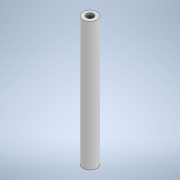
# Autodesk Inventor part: soprye para base bobinas
Saved by Autodesk Inventor 2020 (Build 240168000, 168)
## iProperties
Created: 2022-10-18
Part Number: soprye para base bobinas
Material: Genérico
Document SubType Name: Modeling
Designer: General
Density: 1 g/cm^3
Appearance: Valor por defecto
Author: General
Autodesk Inventor part; units mm, degrees
ref_plane "YZ Plane" through (0, 0, 0) normal (1, 0, 0) x (0, 1, 0)
ref_plane "XZ Plane" through (0, 0, 0) normal (0, 1, 0) x (-1, 0, 0)
ref_plane "XY Plane" through (0, 0, 0) normal (0, 0, 1) x (1, 0, 0)
sketch "Boceto3" plane through (0, 0, 0) normal (0, 1, 0) x (-1, 0, 0)
  circle A0 centre (0, 0) radius 5
  dimension "d10" = 10
  constraints: 1 centre point, 1 coincident
  measures "d10" diameter of A0
extrude "Extrusión2" add sketch "Boceto3" along normal blind 90.7
extrude "Extrusión3" cut sketch "Boceto3" along normal blind 90.7
extrude "Extrusión4" add sketch "Boceto3" along normal blind 90.7
sketch "Boceto4" plane through (0, 90.7, 0) normal (0, 1, 0) x (1, 0, 0)
  point P0 (0, 0)
hole "Agujero2" at (0, 90.7, 0) direction (0, -1, 0) diameter 5 end through all
